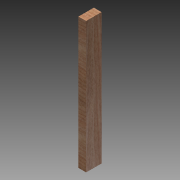
# Autodesk Inventor part: Crossbar
Saved by Autodesk Inventor 2015 SP1 (Build 190203100, 203)
## iProperties
Created: 2015-01-27
Part Number: Crossbar
Material: Generic
Document SubType Name: Modeling
Designer: 55221
Density: 1 g/cm^3
Appearance: Default
Author: 55221
Autodesk Inventor part; units mm, degrees
ref_plane "YZ Plane" through (0, 0, 0) normal (1, 0, 0) x (0, 1, 0)
ref_plane "XZ Plane" through (0, 0, 0) normal (0, 1, 0) x (-1, 0, 0)
ref_plane "XY Plane" through (0, 0, 0) normal (0, 0, 1) x (1, 0, 0)
sketch "Sketch1" plane through (0, 0, 0) normal (1, 0, 0) x (0, 1, 0)
  line L0 (215.9, 25.4) -> (-215.9, 25.4)
  line L1 (-215.9, 25.4) -> (-215.9, -25.4)
  line L2 (-215.9, -25.4) -> (215.9, -25.4)
  line L3 (215.9, -25.4) -> (215.9, 25.4)
  point P0 (0, 0)
  dimension "d0" = 431.8
  dimension "d1" = 50.8
  constraints: 8 end point, 2 parallel, 1 horizontal, 1 perpendicular
  measures "d0" distance of L2.end L1.end
  measures "d1" distance of L1.end L0.end
extrude "Extrusion1" add sketch "Sketch1" along normal blind 25.4
body "Solid1"
